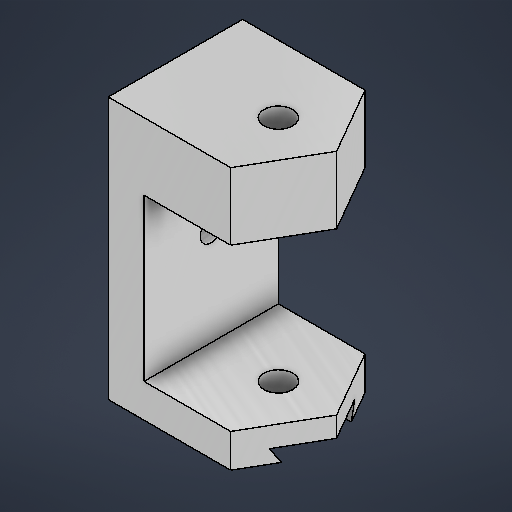
# Autodesk Inventor part: Bearing Sled Single
Saved by Autodesk Inventor 2026 (Build 300175050, 175E)
## iProperties
Created: 2025-05-28
Part Number: Bearing Sled Single
Material: Aluminum 6061
Document SubType Name: Modeling
Designer: Joshua Eah
Density: 2.7 g/cm^3
Appearance: Aluminum - Flat
Author: Joshua Eah
Autodesk Inventor part; units mm, degrees
ref_plane "YZ Plane" through (0, 0, 0) normal (1, 0, 0) x (0, 1, 0)
ref_plane "XZ Plane" through (0, 0, 0) normal (0, 1, 0) x (-1, 0, 0)
ref_plane "XY Plane" through (0, 0, 0) normal (0, 0, 1) x (1, 0, 0)
sketch "Original Profile" plane through (0, 0, 0) normal (0, 1, 0) x (-1, 0, 0)
  line L0 (0, 0) -> (-18, 0)
  line L1 (-18, 0) -> (-18, -15)
  line L2 (-18, -15) -> (0, -15)
  line L3 (0, -15) -> (0, 0)
  line L4 (0, -7.5) -> (-18, -7.5)
  circle A0 centre (-11.5, -7.5) radius 1.5
  circle A1 centre (-11.5, -7.5) radius 6.5
  line L5 (-5, -15) -> (-5, 0)
  line L6 (0, -9.0875) -> (-18, -9.0875)
  line L7 (-18, -9.0875) -> (-18, -5.9125)
  line L8 (-18, -5.9125) -> (0, -5.9125)
  line L9 (0, -5.9125) -> (0, -9.0875)
  point P0 (0, -5.9125)
  point P1 (-18, -9.0875)
  dimension "d8" = 3
  dimension "d9" = 13
  dimension "d10" = 15
  dimension "d11" = 11.5
  dimension "d12" = 6.5
  dimension "d15" = 5
  dimension "d32" = 3.175
  dimension "d33" = 3.175
  constraints: 20 end point, 5 point on line, 4 parallel, 3 perpendicular, 2 centre point, 2 horizontal, 2 midpoint, 1 coincident
  measures "d8" diameter of A0
  measures "d9" diameter of A1
  measures "d10" distance of L2.end L0.start
  measures "d11" distance from line of L3 A0.centre
  measures "d12" distance from line of L1 A0.centre
  measures "d15" distance between parallel lines of L3 L5
  measures "d32" distance between parallel lines of L6 L8
  measures "d33" diameter of L6 L4
extrude "Stock" add sketch "Original Profile" along normal blind 29.25
sketch "Sketch4" plane through (18, 0, 0) normal (1, 0, 0) x (0, 0, -1)
  line L0 (15, 0) -> (15, 29.25) projected
  line L1 (0, 21.75) -> (15, 21.75)
  line L2 (15, 21.75) -> (15, 3.75)
  line L3 (15, 3.75) -> (0, 3.75)
  line L4 (0, 3.75) -> (0, 21.75)
  line L5 (0, 0) -> (0, 29.25) projected
  line L6 (0, 0) -> (15, 0) projected
  line L7 (15, 29.25) -> (0, 29.25) projected
  line L8 (7.5, 29.25) -> (7.5, 0) construction
  line L9 (15, 0) -> (0, 0) projected
  line L10 (2.7375, 0) -> (12.2625, 0)
  line L11 (12.2625, 0) -> (12.2625, 1.5)
  line L12 (12.2625, 1.5) -> (2.7375, 1.5)
  line L13 (2.7375, 1.5) -> (2.7375, 0)
  line L14 (2.7375, 1.5) -> (3.6035, 0)
  line L15 (2.7375, 1.5) -> (4.4696, 1.5) construction
  line L16 (12.2625, 1.5) -> (11.3965, 0)
  line L17 (12.2625, 1.5) -> (13.9946, 1.5) construction
  dimension "d40" = 3.75
  dimension "d41" = 18
  dimension "d44" = 9.525
  dimension "d45" = 4.7625
  dimension "d46" = 1.5
  dimension "d47" = 60
  dimension "d48" = 120
  constraints: 26 end point, 5 point on line, 4 horizontal, 4 parallel, 2 equal length, 2 midpoint, 2 perpendicular
  measures "d40" distance between parallel lines of L3 L6
  measures "d41" distance between parallel lines of L1 L3
  measures "d44" distance of L11.end L12.end
  measures "d45" distance between parallel lines of L8 L13
  measures "d46" distance of L10.end L11.end
  measures "d47" angle of L14 L15
  measures "d48" angle of L16 L17
extrude "Cut Slot" cut sketch "Sketch4" against normal blind 14 contours L3 L4 L1 L0
extrude "Extrusion7" cut sketch "Sketch4" against normal through all contours L6 L14 L12 L16
hole "Hole1" at (11.5, 0, -7.5) direction (0, 1, 0) diameter 3.2004 end through all clearance for "Socket Head Cap Screw" size "M3" standard "Ansi Metric M Profile"
sketch "Sketch5" plane through (0, 0, 0) normal (-1, 0, 0) x (0, 0, 1)
  circle A0 centre (-7.5, 14.625) radius 1.5
  line L0 (-15, 29.25) -> (0, 29.25) projected
  line L1 (-15, 0) -> (-11.3965, 0) projected
  line L2 (-15, 0) -> (-15, 29.25) projected
  point P0 (0, 0)
  dimension "d51" = 3
  dimension "d52" = 14.625
  dimension "d53" = 29.25
  dimension "d54" = 7.5
  constraints: 1 centre point
  measures "d51" diameter of A0
  measures "d52" distance from line of L0 A0.centre
  measures "d53" distance between parallel lines of L1 L0
  measures "d54" distance from line of A0.centre L2
hole "Hole2" at (0, 14.625, -7.5) direction (1, 0, 0) diameter 2.459 end through all thread size "M3x0.5" class "6H" standard "ANSI Metric M Profile"
chamfer "Chamfer1" distance 7.5 angle 30 1 edges at (18, 25.5, 0) measured on face at (18, 24.25, -10)
chamfer "Chamfer2" distance 7.5 angle 30 1 edges at (18, 1.875, 0) measured on face at (18, 3, -5.9125)
chamfer "Chamfer3" distance 7.5 angle 30 1 edges at (18, 25.5, -15) measured on face at (18, 24.25, -10)
chamfer "Chamfer4" distance 7.5 angle 30 1 edges at (18, 1.875, -15) measured on face at (18, 3, -11.5875)
equation "\"d12\" = 0.5 * d9"
equation "\"d33\" = d32"
equation "\"d45\" = 0.5 * d44"
equation "\"d52\" = 0.5 * d53"
body "Solid1"
